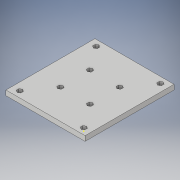
# Autodesk Inventor part: jetson nano mounting plate
Saved by Autodesk Inventor 2019 (Build 230136000, 136)
## iProperties
Created: 2023-11-11
Part Number: jetson nano mounting plate
Material: Generic
Document SubType Name: Modeling
Designer: ony
Density: 1 g/cm^3
Appearance: Default
Author: ony
Autodesk Inventor part; units mm, degrees
ref_plane "YZ Plane" through (0, 0, 0) normal (1, 0, 0) x (0, 1, 0)
ref_plane "XZ Plane" through (0, 0, 0) normal (0, 1, 0) x (-1, 0, 0)
ref_plane "XY Plane" through (0, 0, 0) normal (0, 0, 1) x (1, 0, 0)
sketch "Sketch1" plane through (0, 0, 0) normal (0, 1, 0) x (-1, 0, 0)
  line L0 (0, 0) -> (90, 0)
  line L1 (90, 0) -> (90, -106)
  line L2 (90, -106) -> (0, -106)
  line L3 (0, -106) -> (0, 0)
  dimension "d0" = 106
  dimension "d1" = 90
  constraints: 8 end point, 2 parallel, 1 horizontal, 1 perpendicular
  measures "d0" distance of L0.end L1.end
  measures "d1" distance of L1.end L2.end
extrude "Extrusion1" add sketch "Sketch1" along normal blind 6.35
sketch "Sketch2" plane through (0, 6.35, 0) normal (0, 1, 0) x (1, 0, 0)
  point P0 (0, 0)
sketch "Sketch3" plane through (0, 6.35, 0) normal (0, 1, 0) x (1, 0, 0)
  line L0 (-90, 0) -> (0, 0) projected
  line L1 (0, 0) -> (0, 106) projected
  line L2 (-90, 0) -> (0, 0)
  line L3 (0, 0) -> (0, 106)
  line L4 (0, 106) -> (-90, 106)
  line L5 (-85.94, 3.81) -> (-3.81, 3.81)
  line L6 (-3.81, 3.81) -> (-3.81, 102.19)
  line L7 (-3.81, 102.19) -> (-86.19, 102.19)
  line L8 (-85.94, 3.81) -> (-88.94, 3.81)
  line L9 (-88.94, 5.5421) -> (-85.94, 7.2741)
  line L10 (-85.94, 7.2741) -> (-82.94, 5.5421)
  line L11 (-82.94, 5.5421) -> (-82.94, 2.0779)
  line L12 (-82.94, 2.0779) -> (-85.94, 0.3459)
  line L13 (-85.94, 0.3459) -> (-88.94, 2.0779)
  line L14 (-88.94, 2.0779) -> (-88.94, 5.5421)
  line L15 (-85.69, 102.19) -> (-88.69, 102.19)
  line L16 (-88.69, 103.6334) -> (-86.19, 105.0768)
  line L17 (-86.19, 105.0768) -> (-83.69, 103.6334)
  line L18 (-83.69, 103.6334) -> (-83.69, 100.7466)
  line L19 (-83.69, 100.7466) -> (-86.19, 99.3032)
  line L20 (-86.19, 99.3032) -> (-88.69, 100.7466)
  line L21 (-88.69, 100.7466) -> (-88.69, 103.6334)
  line L22 (-3.31, 102.19) -> (-6.31, 102.19)
  line L23 (-6.31, 103.6334) -> (-3.81, 105.0768)
  line L24 (-3.81, 105.0768) -> (-1.31, 103.6334)
  line L25 (-1.31, 103.6334) -> (-1.31, 100.7466)
  line L26 (-1.31, 100.7466) -> (-3.81, 99.3032)
  line L27 (-3.81, 99.3032) -> (-6.31, 100.7466)
  line L28 (-6.31, 100.7466) -> (-6.31, 103.6334)
  line L29 (-3.31, 3.81) -> (-6.31, 3.81)
  line L30 (-6.31, 5.2534) -> (-3.81, 6.6968)
  line L31 (-3.81, 6.6968) -> (-1.31, 5.2534)
  line L32 (-1.31, 5.2534) -> (-1.31, 2.3666)
  line L33 (-1.31, 2.3666) -> (-3.81, 0.9232)
  line L34 (-3.81, 0.9232) -> (-6.31, 2.3666)
  line L35 (-6.31, 2.3666) -> (-6.31, 5.2534)
  dimension "d5" = 3
  dimension "d6" = 3
  dimension "d7" = 3
  dimension "d8" = 3
  constraints: 68 end point, 5 horizontal, 4 midpoint, 2 parallel, 2 perpendicular, 1 coincident, 15 other
  measures "d5" distance of L5.start L8.end
  measures "d6" distance of L15.start L15.end
  measures "d7" distance of L22.start L22.end
  measures "d8" distance of L29.start L29.end
extrude "Extrusion2" cut sketch "Sketch3" against normal blind 6.35
sketch "Sketch4" plane through (0, 6.35, 0) normal (0, 1, 0) x (1, 0, 0)
  line L0 (0, 0) -> (-90, 0) projected
  line L1 (-45, 0) -> (-45, 106)
  line L2 (0, 106) -> (-90, 106) projected
  line L3 (5.8, -4.15) -> (-95.8, -4.15)
  line L4 (-95.8, -4.15) -> (-95.8, 110.15)
  line L5 (-95.8, 110.15) -> (5.8, 110.15)
  line L6 (5.8, 110.15) -> (5.8, -4.15)
  line L7 (5.8, -4.15) -> (-95.8, 110.15) construction
  line L8 (-95.8, -4.15) -> (5.8, 110.15) construction
  line L9 (-90, 0) -> (0, 0)
  line L10 (0, 0) -> (0, 106)
  line L11 (0, 106) -> (-90, 106)
  line L12 (-90, 106) -> (-90, 0)
  point P0 (-45, 53)
  dimension "d11" = 101.6
  dimension "d12" = 114.3
  constraints: 22 end point, 5 midpoint, 4 parallel, 2 horizontal, 2 perpendicular
  measures "d11" distance of L4.end L5.end
  measures "d12" distance of L3.end L4.end
extrude "Extrusion3" add sketch "Sketch4" against normal blind 6.35
sketch "Sketch5" plane through (0, 6.35, 0) normal (0, 1, 0) x (1, 0, 0)
  line L0 (-90, 0) -> (0, 0)
  line L1 (0, 0) -> (0, 106)
  line L2 (-90, 0) -> (0, 0)
  line L3 (0, 0) -> (0, 106)
  line L4 (0, 106) -> (-90, 106)
  line L5 (-85.94, 3.81) -> (-3.81, 3.81)
  line L6 (-3.81, 3.81) -> (-3.81, 102.19)
  line L7 (-3.81, 102.19) -> (-86.19, 102.19)
  line L8 (-85.94, 3.81) -> (-88.94, 3.81)
  line L9 (-88.94, 5.5421) -> (-85.94, 7.2741)
  line L10 (-85.94, 7.2741) -> (-82.94, 5.5421)
  line L11 (-82.94, 5.5421) -> (-82.94, 2.0779)
  line L12 (-82.94, 2.0779) -> (-85.94, 0.3459)
  line L13 (-85.94, 0.3459) -> (-88.94, 2.0779)
  line L14 (-88.94, 2.0779) -> (-88.94, 5.5421)
  line L15 (-86.19, 99.3032) -> (-88.69, 100.7466)
  line L16 (-83.69, 100.7466) -> (-86.19, 99.3032)
  line L17 (-86.19, 102.19) -> (-88.69, 102.19)
  line L18 (-88.69, 100.7466) -> (-88.69, 103.6334)
  line L19 (-88.69, 103.6334) -> (-86.19, 105.0768)
  line L20 (-86.19, 105.0768) -> (-83.69, 103.6334)
  line L21 (-83.69, 103.6334) -> (-83.69, 100.7466)
  line L22 (-3.81, 99.3032) -> (-6.31, 100.7466)
  line L23 (-1.31, 100.7466) -> (-3.81, 99.3032)
  line L24 (-3.81, 102.19) -> (-6.31, 102.19)
  line L25 (-6.31, 100.7466) -> (-6.31, 103.6334)
  line L26 (-6.31, 103.6334) -> (-3.81, 105.0768)
  line L27 (-3.81, 105.0768) -> (-1.31, 103.6334)
  line L28 (-1.31, 103.6334) -> (-1.31, 100.7466)
  line L29 (-3.81, 0.9232) -> (-6.31, 2.3666)
  line L30 (-1.31, 2.3666) -> (-3.81, 0.9232)
  line L31 (-3.81, 3.81) -> (-6.31, 3.81)
  line L32 (-6.31, 2.3666) -> (-6.31, 5.2534)
  line L33 (-6.31, 5.2534) -> (-3.81, 6.6968)
  line L34 (-3.81, 6.6968) -> (-1.31, 5.2534)
  line L35 (-1.31, 5.2534) -> (-1.31, 2.3666)
  line L36 (5.8, -4.15) -> (-95.8, -4.15) projected
  line L37 (-45, -4.15) -> (-45, 110.15)
  line L38 (-95.8, 110.15) -> (5.8, 110.15) projected
  line L39 (-25.95, 33.95) -> (-64.05, 33.95)
  line L40 (-64.05, 33.95) -> (-64.05, 72.05)
  line L41 (-64.05, 72.05) -> (-25.95, 72.05)
  line L42 (-25.95, 72.05) -> (-25.95, 33.95)
  line L43 (-25.95, 33.95) -> (-64.05, 72.05) construction
  line L44 (-64.05, 33.95) -> (-25.95, 72.05) construction
  line L45 (-63.55, 33.95) -> (-66.55, 33.95)
  line L46 (-66.55, 35.3934) -> (-64.05, 36.8368)
  line L47 (-64.05, 36.8368) -> (-61.55, 35.3934)
  line L48 (-61.55, 35.3934) -> (-61.55, 32.5066)
  line L49 (-61.55, 32.5066) -> (-64.05, 31.0632)
  line L50 (-64.05, 31.0632) -> (-66.55, 32.5066)
  line L51 (-66.55, 32.5066) -> (-66.55, 35.3934)
  line L52 (-63.55, 72.05) -> (-66.55, 72.05)
  line L53 (-66.55, 73.4934) -> (-64.05, 74.9368)
  line L54 (-64.05, 74.9368) -> (-61.55, 73.4934)
  line L55 (-61.55, 73.4934) -> (-61.55, 70.6066)
  line L56 (-61.55, 70.6066) -> (-64.05, 69.1632)
  line L57 (-64.05, 69.1632) -> (-66.55, 70.6066)
  line L58 (-66.55, 70.6066) -> (-66.55, 73.4934)
  line L59 (-25.45, 33.95) -> (-28.45, 33.95)
  line L60 (-28.45, 35.3934) -> (-25.95, 36.8368)
  line L61 (-25.95, 36.8368) -> (-23.45, 35.3934)
  line L62 (-23.45, 35.3934) -> (-23.45, 32.5066)
  line L63 (-23.45, 32.5066) -> (-25.95, 31.0632)
  line L64 (-25.95, 31.0632) -> (-28.45, 32.5066)
  line L65 (-28.45, 32.5066) -> (-28.45, 35.3934)
  line L66 (-25.45, 72.05) -> (-28.45, 72.05)
  line L67 (-28.45, 73.4934) -> (-25.95, 74.9368)
  line L68 (-25.95, 74.9368) -> (-23.45, 73.4934)
  line L69 (-23.45, 73.4934) -> (-23.45, 70.6066)
  line L70 (-23.45, 70.6066) -> (-25.95, 69.1632)
  line L71 (-25.95, 69.1632) -> (-28.45, 70.6066)
  line L72 (-28.45, 70.6066) -> (-28.45, 73.4934)
  point P0 (-45, 53)
  dimension "d15" = 3
  dimension "d16" = 2.5
  dimension "d17" = 2.5
  dimension "d18" = 2.5
  dimension "d19" = 38.1
  dimension "d20" = 38.1
  dimension "d21" = 3
  dimension "d22" = 3
  dimension "d23" = 3
  dimension "d24" = 3
  constraints: 142 end point, 13 midpoint, 10 horizontal, 4 parallel, 3 perpendicular, 1 coincident, 15 other
  measures "d15" distance of L5.start L8.end
  measures "d16" distance of L17.start L17.end
  measures "d17" distance of L24.start L24.end
  measures "d18" distance of L31.start L31.end
  measures "d19" distance of L40.end L41.end
  measures "d20" distance of L39.end L40.end
  measures "d21" distance of L45.start L45.end
  measures "d22" distance of L52.start L52.end
  measures "d23" distance of L59.start L59.end
  measures "d24" distance of L66.start L66.end
extrude "Extrusion4" cut sketch "Sketch5" against normal blind 6.35 contours L65 L60 L42 L39 | L39 L42 L61 L62 L63 L64 L65 | L48 L49 L50 L51 L45 L39 | L39 L40 L47 L48 | L55 L56 L40 L41 | L41 L52 L58 L53 L54 L55 | L72 L67 L68 L69 L70 L42 L41 | L41 L42 L71 L72 | L45 L51 L46 L40 | L40 L57 L58 L52
sketch "Sketch6" plane through (0, 6.35, 0) normal (0, 1, 0) x (1, 0, 0)
  point P0 (0, 0)
sketch "Sketch7" plane through (0, 6.35, 0) normal (0, 1, 0) x (1, 0, 0)
  line L0 (-64.05, 33.95) -> (-67.05, 33.95)
  line L1 (-67.05, 35.6821) -> (-64.05, 37.4141)
  line L2 (-64.05, 37.4141) -> (-61.05, 35.6821)
  line L3 (-61.05, 35.6821) -> (-61.05, 32.2179)
  line L4 (-61.05, 32.2179) -> (-64.05, 30.4859)
  line L5 (-64.05, 30.4859) -> (-67.05, 32.2179)
  line L6 (-67.05, 32.2179) -> (-67.05, 35.6821)
  line L7 (-64.05, 69.1632) -> (-66.55, 70.6066) projected
  line L8 (-64.05, 74.9368) -> (-61.55, 73.4934) projected
  line L9 (-25.95, 31.0632) -> (-23.45, 32.5066) projected
  line L10 (-23.45, 35.3934) -> (-25.95, 36.8368) projected
  line L11 (-28.45, 70.6066) -> (-25.95, 69.1632) projected
  line L12 (-61.55, 70.6066) -> (-64.05, 69.1632) projected
  line L13 (-64.05, 69.1632) -> (-64.05, 72.05)
  line L14 (-28.45, 32.5066) -> (-25.95, 31.0632) projected
  line L15 (-25.95, 31.0632) -> (-25.95, 33.95)
  line L16 (-25.95, 69.1632) -> (-25.95, 72.05)
  line L17 (-64.05, 72.05) -> (-67.05, 72.05)
  line L18 (-67.05, 73.7821) -> (-64.05, 75.5141)
  line L19 (-64.05, 75.5141) -> (-61.05, 73.7821)
  line L20 (-61.05, 73.7821) -> (-61.05, 70.3179)
  line L21 (-61.05, 70.3179) -> (-64.05, 68.5859)
  line L22 (-64.05, 68.5859) -> (-67.05, 70.3179)
  line L23 (-67.05, 70.3179) -> (-67.05, 73.7821)
  line L24 (-25.95, 72.05) -> (-28.95, 72.05)
  line L25 (-28.95, 73.7821) -> (-25.95, 75.5141)
  line L26 (-25.95, 75.5141) -> (-22.95, 73.7821)
  line L27 (-22.95, 73.7821) -> (-22.95, 70.3179)
  line L28 (-22.95, 70.3179) -> (-25.95, 68.5859)
  line L29 (-25.95, 68.5859) -> (-28.95, 70.3179)
  line L30 (-28.95, 70.3179) -> (-28.95, 73.7821)
  line L31 (-25.95, 33.95) -> (-28.95, 33.95)
  line L32 (-28.95, 35.6821) -> (-25.95, 37.4141)
  line L33 (-25.95, 37.4141) -> (-22.95, 35.6821)
  line L34 (-22.95, 35.6821) -> (-22.95, 32.2179)
  line L35 (-22.95, 32.2179) -> (-25.95, 30.4859)
  line L36 (-25.95, 30.4859) -> (-28.95, 32.2179)
  line L37 (-28.95, 32.2179) -> (-28.95, 35.6821)
  line L38 (-85.94, 7.2741) -> (-82.94, 5.5421) projected
  line L39 (-85.94, 0.3459) -> (-85.94, 7.2741)
  line L40 (-85.94, 3.81) -> (-88.94, 3.81)
  line L41 (-88.94, 5.5421) -> (-88.94, 2.0779) projected
  line L42 (-85.94, 3.81) -> (-88.94, 3.81)
  line L43 (-88.94, 5.5421) -> (-85.94, 7.2741)
  line L44 (-85.94, 7.2741) -> (-82.94, 5.5421)
  line L45 (-82.94, 5.5421) -> (-82.94, 2.0779)
  line L46 (-82.94, 2.0779) -> (-85.94, 0.3459)
  line L47 (-85.94, 0.3459) -> (-88.94, 2.0779)
  line L48 (-88.94, 2.0779) -> (-88.94, 5.5421)
  line L49 (-3.81, 0.9232) -> (-1.31, 2.3666) projected
  line L50 (-3.81, 0.9232) -> (-3.81, 3.81)
  line L51 (-1.31, 100.7466) -> (-3.81, 99.3032) projected
  line L52 (-3.81, 105.0768) -> (-6.31, 103.6334) projected
  line L53 (-3.81, 99.3032) -> (-3.81, 102.19)
  line L54 (-3.81, 102.19) -> (-6.81, 102.19)
  line L55 (-6.81, 103.9221) -> (-3.81, 105.6541)
  line L56 (-3.81, 105.6541) -> (-0.81, 103.9221)
  line L57 (-0.81, 103.9221) -> (-0.81, 100.4579)
  line L58 (-0.81, 100.4579) -> (-3.81, 98.7259)
  line L59 (-3.81, 98.7259) -> (-6.81, 100.4579)
  line L60 (-6.81, 100.4579) -> (-6.81, 103.9221)
  line L61 (-3.81, 3.81) -> (-6.81, 3.81)
  line L62 (-6.81, 5.5421) -> (-3.81, 7.2741)
  line L63 (-3.81, 7.2741) -> (-0.81, 5.5421)
  line L64 (-0.81, 5.5421) -> (-0.81, 2.0779)
  line L65 (-0.81, 2.0779) -> (-3.81, 0.3459)
  line L66 (-3.81, 0.3459) -> (-6.81, 2.0779)
  line L67 (-6.81, 2.0779) -> (-6.81, 5.5421)
  point P0 (0, 0)
  point P1 (-64.05, 36.8368)
  point P2 (-3.81, 6.6968)
  constraints: 112 end point, 9 midpoint, 7 coincident, 7 horizontal, 1 vertical, 91 other
extrude "Extrusion5" cut sketch "Sketch7" against normal blind 6.35 contours L1 L2 L3 L4 L5 L6 | L18 L19 L20 L21 L22 L23 | L25 L26 L27 L28 L29 L30 | L32 L33 L34 L35 L36 L37
sketch "Sketch8" plane through (0, 6.35, 0) normal (0, 1, 0) x (1, 0, 0)
  line L0 (-64.05, 33.95) -> (-67.05, 33.95)
  line L1 (-67.05, 35.6821) -> (-64.05, 37.4141)
  line L2 (-64.05, 37.4141) -> (-61.05, 35.6821)
  line L3 (-61.05, 35.6821) -> (-61.05, 32.2179)
  line L4 (-61.05, 32.2179) -> (-64.05, 30.4859)
  line L5 (-64.05, 30.4859) -> (-67.05, 32.2179)
  line L6 (-67.05, 32.2179) -> (-67.05, 35.6821)
  line L7 (-25.95, 31.0632) -> (-23.45, 32.5066)
  line L8 (-23.45, 35.3934) -> (-25.95, 36.8368)
  line L9 (-28.45, 70.6066) -> (-25.95, 69.1632)
  line L10 (-64.05, 69.1632) -> (-64.05, 72.05)
  line L11 (-28.45, 32.5066) -> (-25.95, 31.0632)
  line L12 (-25.95, 31.0632) -> (-25.95, 33.95)
  line L13 (-25.95, 69.1632) -> (-25.95, 72.05)
  line L14 (-64.05, 72.05) -> (-67.05, 72.05)
  line L15 (-61.05, 73.7821) -> (-61.05, 70.3179)
  line L16 (-64.05, 75.5141) -> (-61.05, 73.7821)
  line L17 (-61.05, 70.3179) -> (-64.05, 68.5859)
  line L18 (-67.05, 73.7821) -> (-64.05, 75.5141)
  line L19 (-67.05, 70.3179) -> (-67.05, 73.7821)
  line L20 (-64.05, 68.5859) -> (-67.05, 70.3179)
  line L21 (-25.95, 72.05) -> (-28.95, 72.05)
  line L22 (-22.95, 73.7821) -> (-22.95, 70.3179)
  line L23 (-25.95, 75.5141) -> (-22.95, 73.7821)
  line L24 (-22.95, 70.3179) -> (-25.95, 68.5859)
  line L25 (-28.95, 73.7821) -> (-25.95, 75.5141)
  line L26 (-28.95, 70.3179) -> (-28.95, 73.7821)
  line L27 (-25.95, 68.5859) -> (-28.95, 70.3179)
  line L28 (-25.95, 33.95) -> (-28.95, 33.95)
  line L29 (-22.95, 35.6821) -> (-22.95, 32.2179)
  line L30 (-25.95, 37.4141) -> (-22.95, 35.6821)
  line L31 (-22.95, 32.2179) -> (-25.95, 30.4859)
  line L32 (-28.95, 35.6821) -> (-25.95, 37.4141)
  line L33 (-28.95, 32.2179) -> (-28.95, 35.6821)
  line L34 (-25.95, 30.4859) -> (-28.95, 32.2179)
  line L35 (-85.94, 7.2741) -> (-82.94, 5.5421)
  line L36 (-85.94, 0.3459) -> (-85.94, 7.2741)
  line L37 (-85.94, 3.81) -> (-88.94, 3.81)
  line L38 (-88.94, 5.5421) -> (-88.94, 2.0779)
  line L39 (-85.94, 3.81) -> (-88.94, 3.81)
  line L40 (-88.94, 5.5421) -> (-85.94, 7.2741)
  line L41 (-85.94, 7.2741) -> (-82.94, 5.5421)
  line L42 (-82.94, 5.5421) -> (-82.94, 2.0779)
  line L43 (-82.94, 2.0779) -> (-85.94, 0.3459)
  line L44 (-85.94, 0.3459) -> (-88.94, 2.0779)
  line L45 (-88.94, 2.0779) -> (-88.94, 5.5421)
  line L46 (-3.81, 0.9232) -> (-1.31, 2.3666)
  line L47 (-3.81, 0.9232) -> (-3.81, 3.81)
  line L48 (-1.31, 100.7466) -> (-3.81, 99.3032)
  line L49 (-3.81, 105.0768) -> (-6.31, 103.6334)
  line L50 (-3.81, 99.3032) -> (-3.81, 102.19)
  line L51 (-3.81, 102.19) -> (-6.81, 102.19)
  line L52 (-0.81, 103.9221) -> (-0.81, 100.4579)
  line L53 (-0.81, 100.4579) -> (-3.81, 98.7259)
  line L54 (-3.81, 105.6541) -> (-0.81, 103.9221)
  line L55 (-6.81, 103.9221) -> (-3.81, 105.6541)
  line L56 (-6.81, 100.4579) -> (-6.81, 103.9221)
  line L57 (-3.81, 98.7259) -> (-6.81, 100.4579)
  line L58 (-3.81, 3.81) -> (-6.81, 3.81)
  line L59 (-0.81, 5.5421) -> (-0.81, 2.0779)
  line L60 (-0.81, 2.0779) -> (-3.81, 0.3459)
  line L61 (-3.81, 7.2741) -> (-0.81, 5.5421)
  line L62 (-6.81, 5.5421) -> (-3.81, 7.2741)
  line L63 (-6.81, 2.0779) -> (-6.81, 5.5421)
  line L64 (-3.81, 0.3459) -> (-6.81, 2.0779)
  line L65 (-67.05, 70.3179) -> (-64.05, 68.5859) projected
  line L66 (-64.05, 69.1632) -> (-64.05, 68.5859)
  line L67 (-86.19, 99.3032) -> (-83.69, 100.7466) projected
  line L68 (-86.19, 105.0768) -> (-86.19, 102.19)
  line L69 (-83.69, 100.7466) -> (-86.19, 99.3032)
  line L70 (-86.19, 105.0768) -> (-88.69, 103.6334)
  line L71 (-86.19, 99.3032) -> (-86.19, 102.19)
  line L72 (-86.19, 102.19) -> (-89.19, 102.19)
  line L73 (-83.19, 103.9221) -> (-83.19, 100.4579)
  line L74 (-83.19, 100.4579) -> (-86.19, 98.7259)
  line L75 (-86.19, 105.6541) -> (-83.19, 103.9221)
  line L76 (-89.19, 103.9221) -> (-86.19, 105.6541)
  line L77 (-89.19, 100.4579) -> (-89.19, 103.9221)
  line L78 (-86.19, 98.7259) -> (-89.19, 100.4579)
  point P0 (0, 0)
  point P1 (0, 0)
  point P2 (-64.05, 36.8368)
  point P3 (-3.81, 6.6968)
  constraints: 154 end point, 10 midpoint, 8 coincident, 8 horizontal, 2 vertical, 104 other
extrude "Extrusion6" cut sketch "Sketch8" against normal blind 25.4
body "Solid1"
